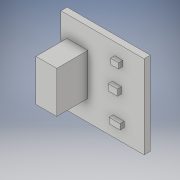
# Autodesk Inventor part: sunlightsensor
Saved by Autodesk Inventor 2019 (Build 230136000, 136)
## iProperties
Created: 2018-06-16
Part Number: sunlightsensor
Material: Generic
Document SubType Name: Modeling
Designer: daniel
Density: 1 g/cm^3
Appearance: Default
Author: daniel
Autodesk Inventor part; units mm, degrees
ref_plane "YZ Plane" through (0, 0, 0) normal (1, 0, 0) x (0, 1, 0)
ref_plane "XZ Plane" through (0, 0, 0) normal (0, 1, 0) x (-1, 0, 0)
ref_plane "XY Plane" through (0, 0, 0) normal (0, 0, 1) x (1, 0, 0)
sketch "Sketch1" plane through (0, 0, 0) normal (0, 0, 1) x (1, 0, 0)
  line L0 (-10, -10) -> (10, -10)
  line L1 (10, -10) -> (10, 10)
  line L2 (10, 10) -> (-10, 10)
  line L3 (-10, 10) -> (-10, -10)
  line L4 (-10, -10) -> (10, 10) construction
  line L5 (10, -10) -> (-10, 10) construction
  point P0 (0, 0)
  dimension "d0" = 20
  dimension "d1" = 20
  constraints: 12 end point, 2 midpoint, 2 parallel, 1 horizontal, 1 perpendicular
  measures "d0" distance of L2.end L1.end
  measures "d1" distance of L1.end L0.end
extrude "Extrusion1" add sketch "Sketch1" along normal blind 1.5
sketch "Sketch2" plane through (0, 0, 1.5) normal (0, 0, 1) x (1, 0, 0)
  line L0 (-14, 0) -> (14, 0) projected
  line L1 (-8.5, -5) -> (-3.5, -5)
  line L2 (-3.5, -5) -> (-3.5, 5)
  line L3 (-3.5, 5) -> (-8.5, 5)
  line L4 (-8.5, 5) -> (-8.5, -5)
  line L5 (-8.5, -5) -> (-3.5, 5) construction
  line L6 (-3.5, -5) -> (-8.5, 5) construction
  line L7 (-10, 10) -> (-10, -10) projected
  point P0 (0, 0)
  point P1 (-6, 0)
  dimension "d4" = 1.5
  dimension "d5" = 10
  dimension "d6" = 5
  constraints: 12 end point, 2 midpoint, 2 parallel, 1 horizontal, 1 perpendicular, 1 point on line
  measures "d4" distance between parallel lines of L7 L4
  measures "d5" distance of L1.end L2.end
  measures "d6" distance of L2.end L3.end
extrude "Extrusion2" add sketch "Sketch2" along normal blind 7.5
sketch "Sketch3" plane through (0, 0, 1.5) normal (0, 0, 1) x (1, 0, 0)
  line L0 (2.9488, 7.102) -> (4.8593, 7.102)
  line L1 (4.8593, 7.102) -> (4.8593, 5.773)
  line L2 (4.8593, 5.773) -> (2.9488, 5.773)
  line L3 (2.9488, 5.773) -> (2.9488, 7.102)
  line L4 (2.9488, 7.102) -> (4.8593, 5.773) construction
  line L5 (4.8593, 7.102) -> (2.9488, 5.773) construction
  line L6 (2.3673, 1.4952) -> (4.6101, 1.4952)
  line L7 (4.6101, 1.4952) -> (4.6101, 0)
  line L8 (4.6101, 0) -> (2.3673, 0)
  line L9 (2.3673, 0) -> (2.3673, 1.4952)
  line L10 (2.3673, 1.4952) -> (4.6101, 0) construction
  line L11 (4.6101, 1.4952) -> (2.3673, 0) construction
  line L12 (2.575, -5.3992) -> (5.233, -5.3992)
  line L13 (5.233, -5.3992) -> (5.233, -6.7282)
  line L14 (5.233, -6.7282) -> (2.575, -6.7282)
  line L15 (2.575, -6.7282) -> (2.575, -5.3992)
  line L16 (2.575, -5.3992) -> (5.233, -6.7282) construction
  line L17 (5.233, -5.3992) -> (2.575, -6.7282) construction
  point P0 (0, 0)
  point P1 (3.904, 6.4375)
  point P2 (3.4887, 0.7476)
  point P3 (3.904, -6.0637)
  constraints: 36 end point, 6 midpoint, 6 parallel, 3 horizontal, 3 perpendicular
extrude "Extrusion3" add sketch "Sketch3" along normal blind 1
body "Solid1"
